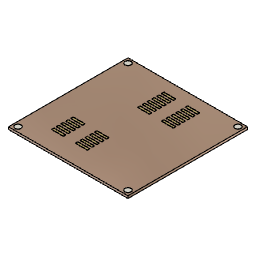
Placa v4 (Autodesk Fusion 360 design; units mm, degrees)
Autodesk Fusion 360 part; units mm, degrees
form "Form1" [no effect]
sketch "SketchPlaca" plane through (0, 0, 0) normal (0, 1, 0) x (1, 0, 0)
  line L0 (0, 0) -> (50, 0)
  line L1 (50, 0) -> (50, -50)
  line L2 (50, -50) -> (0, -50)
  line L3 (0, -50) -> (0, 0)
  dimension "d97" = 50
  dimension "d98" = 50
  constraint horizontal L0
  constraint vertical L1
  constraint horizontal L2
  constraint vertical L3
  constraint coincident L0.start L3.end
  measures "d97" distance of L0.start L0.end
  measures "d98" distance of L0.start L2.end
extrude "Extrude39" add sketch "SketchPlaca" along normal blind 1 makes body 1
sketch "SketchHoyos" plane through (0, 0, 0) normal (0, -1, 0) x (1, 0, 0)
  line L0 (50, 50) -> (0, 50)
  line L1 (0, 50) -> (0, 0)
  line L2 (0, 0) -> (50, 0)
  line L3 (50, 0) -> (50, 50)
  circle A0 centre (2, 48) radius 1.25
  circle A1 centre (2, 2) radius 1.25
  circle A2 centre (48, 2) radius 1.25
  circle A3 centre (48, 48) radius 1.25
  line L4 (1.3017, 49.0368) -> (2.7, 46.9644)
  line L5 (2.8637, 48.9036) -> (1.1304, 47.102)
  line L6 (1.1304, 2.898) -> (2.8637, 1.0964)
  line L7 (1.1827, 1.0542) -> (2.8245, 2.9395)
  line L8 (47.1174, 2.8852) -> (48.8811, 1.1134)
  line L9 (48.7554, 2.9959) -> (47.2457, 1.0032)
  line L10 (46.8338, 48.45) -> (49.1623, 47.5401)
  line L11 (48.285, 49.2171) -> (47.7194, 46.7819)
  dimension "d101" = 2.5
  dimension "d102" = 2.5
  dimension "d103" = 2.5
  dimension "d104" = 2.5
  constraint coincident A0 L4.start
  constraint coincident A0 L4.end
  constraint coincident A0 L5.start
  constraint coincident A0 L5.end
  constraint coincident A1 L6.start
  constraint coincident A1 L6.end
  constraint coincident A1 L7.start
  constraint coincident A1 L7.end
  constraint coincident A2 L8.start
  constraint coincident A2 L8.end
  constraint coincident A2 L9.start
  constraint coincident A2 L9.end
  constraint coincident A3 L10.start
  constraint coincident A3 L10.end
  constraint coincident A3 L11.start
  constraint coincident A3 L11.end
  measures "d101" diameter of A0
  measures "d102" diameter of A1
  measures "d103" diameter of A2
  measures "d104" diameter of A3
extrude "Extrude40" add sketch "SketchHoyos" along normal blind 0.1 separate body contours A0 L4 L5 | A0 L4 L5 | A0 L4 L5 | A0 L4 L5 makes body 2
extrude "Extrude41" add sketch "SketchHoyos" along normal blind 0.1 separate body contours A1 L6 L7 | A1 L6 L7 | A1 L6 L7 | A1 L6 L7 makes body 3
extrude "Extrude42" add sketch "SketchHoyos" along normal blind 0.1 separate body contours A2 L8 L9 | A2 L8 L9 | A2 L8 L9 | A2 L8 L9 makes body 4
extrude "Extrude43" add sketch "SketchHoyos" along normal blind 0.1 separate body contours A3 L10 L11 | A3 L10 L11 | A3 L10 L11 | A3 L10 L11 makes body 5
sketch "SketchPaths" plane through (0, 0, 0) normal (0, -1, 0) x (1, 0, 0)
  line L0 (50, 50) -> (0, 50)
  line L1 (0, 50) -> (0, 0)
  line L2 (0, 0) -> (50, 0)
  line L3 (50, 0) -> (50, 50)
  line L4 (10, 15) -> (15, 15)
  line L5 (15, 15) -> (15, 14)
  line L6 (15, 14) -> (10, 14)
  line L7 (10, 14) -> (10, 15)
  line L8 (10, 13) -> (15, 13)
  line L9 (15, 13) -> (15, 12)
  line L10 (15, 12) -> (10, 12)
  line L11 (10, 12) -> (10, 13)
  line L12 (10, 11) -> (15, 11)
  line L13 (15, 11) -> (15, 10)
  line L14 (15, 10) -> (10, 10)
  line L15 (10, 10) -> (10, 11)
  line L16 (10, 9) -> (15, 9)
  line L17 (15, 9) -> (15, 8)
  line L18 (15, 8) -> (10, 8)
  line L19 (10, 8) -> (10, 9)
  line L20 (10, 17) -> (15, 17)
  line L21 (15, 17) -> (15, 16)
  line L22 (15, 16) -> (10, 16)
  line L23 (10, 16) -> (10, 17)
  line L24 (20, 17) -> (25, 17)
  line L25 (25, 17) -> (25, 16)
  line L26 (25, 16) -> (20, 16)
  line L27 (20, 16) -> (20, 17)
  line L28 (20, 15) -> (25, 15)
  line L29 (25, 15) -> (25, 14)
  line L30 (25, 14) -> (20, 14)
  line L31 (20, 14) -> (20, 15)
  line L32 (20, 13) -> (25, 13)
  line L33 (25, 13) -> (25, 12)
  line L34 (25, 12) -> (20, 12)
  line L35 (20, 12) -> (20, 13)
  line L36 (20, 11) -> (25, 11)
  line L37 (25, 11) -> (25, 10)
  line L38 (25, 10) -> (20, 10)
  line L39 (20, 10) -> (20, 11)
  line L40 (20, 9) -> (25, 9)
  line L41 (25, 9) -> (25, 8)
  line L42 (25, 8) -> (20, 8)
  line L43 (20, 8) -> (20, 9)
  line L44 (20, 45) -> (25, 45)
  line L45 (25, 45) -> (25, 44)
  line L46 (25, 44) -> (20, 44)
  line L47 (20, 44) -> (20, 45)
  line L48 (20, 43) -> (25, 43)
  line L49 (25, 43) -> (25, 42)
  line L50 (25, 42) -> (20, 42)
  line L51 (20, 42) -> (20, 43)
  line L52 (20, 41) -> (25, 41)
  line L53 (25, 41) -> (25, 40)
  line L54 (25, 40) -> (20, 40)
  line L55 (20, 40) -> (20, 41)
  line L56 (20, 39) -> (25, 39)
  line L57 (25, 39) -> (25, 38)
  line L58 (25, 38) -> (20, 38)
  line L59 (20, 38) -> (20, 39)
  line L60 (20, 37) -> (25, 37)
  line L61 (25, 37) -> (25, 36)
  line L62 (25, 36) -> (20, 36)
  line L63 (20, 36) -> (20, 37)
  line L64 (20, 35) -> (25, 35)
  line L65 (25, 35) -> (25, 34)
  line L66 (25, 34) -> (20, 34)
  line L67 (20, 34) -> (20, 35)
  line L68 (30, 45) -> (35, 45)
  line L69 (35, 45) -> (35, 44)
  line L70 (35, 44) -> (30, 44)
  line L71 (30, 44) -> (30, 45)
  line L72 (30, 43) -> (35, 43)
  line L73 (35, 43) -> (35, 42)
  line L74 (35, 42) -> (30, 42)
  line L75 (30, 42) -> (30, 43)
  line L76 (30, 41) -> (35, 41)
  line L77 (35, 41) -> (35, 40)
  line L78 (35, 40) -> (30, 40)
  line L79 (30, 40) -> (30, 41)
  line L80 (30, 39) -> (35, 39)
  line L81 (35, 39) -> (35, 38)
  line L82 (35, 38) -> (30, 38)
  line L83 (30, 38) -> (30, 39)
  line L84 (30, 37) -> (35, 37)
  line L85 (35, 37) -> (35, 36)
  line L86 (35, 36) -> (30, 36)
  line L87 (30, 36) -> (30, 37)
  line L88 (30, 35) -> (35, 35)
  line L89 (35, 35) -> (35, 34)
  line L90 (35, 34) -> (30, 34)
  line L91 (30, 34) -> (30, 35)
  dimension "d114" = 1
  constraint horizontal L4
  constraint vertical L5
  constraint horizontal L6
  constraint vertical L7
  constraint horizontal L8
  constraint vertical L9
  constraint horizontal L10
  constraint vertical L11
  constraint horizontal L12
  constraint vertical L13
  constraint horizontal L14
  constraint vertical L15
  constraint horizontal L16
  constraint vertical L17
  constraint horizontal L18
  constraint vertical L19
  constraint horizontal L20
  constraint vertical L21
  constraint horizontal L22
  constraint vertical L23
  constraint horizontal L24
  constraint vertical L25
  constraint horizontal L26
  constraint vertical L27
  constraint horizontal L28
  constraint vertical L29
  constraint horizontal L30
  constraint vertical L31
  constraint horizontal L32
  constraint vertical L33
  constraint horizontal L34
  constraint vertical L35
  constraint horizontal L36
  constraint vertical L37
  constraint horizontal L38
  constraint vertical L39
  constraint horizontal L40
  constraint vertical L41
  constraint horizontal L42
  constraint vertical L43
  constraint horizontal L44
  constraint vertical L45
  constraint horizontal L46
  constraint vertical L47
  constraint horizontal L48
  constraint vertical L49
  constraint horizontal L50
  constraint vertical L51
  constraint horizontal L52
  constraint vertical L53
  constraint horizontal L54
  constraint vertical L55
  constraint horizontal L56
  constraint vertical L57
  constraint horizontal L58
  constraint vertical L59
  constraint horizontal L60
  constraint vertical L61
  constraint horizontal L62
  constraint vertical L63
  constraint horizontal L64
  constraint vertical L65
  constraint horizontal L66
  constraint vertical L67
  constraint horizontal L68
  constraint vertical L69
  constraint horizontal L70
  constraint vertical L71
  constraint horizontal L72
  constraint vertical L73
  constraint horizontal L74
  constraint vertical L75
  constraint horizontal L76
  constraint vertical L77
  constraint horizontal L78
  constraint vertical L79
  constraint horizontal L80
  constraint vertical L81
  constraint horizontal L82
  constraint vertical L83
  constraint horizontal L84
  constraint vertical L85
  constraint horizontal L86
  constraint vertical L87
  constraint horizontal L88
  constraint vertical L89
  constraint horizontal L90
  constraint vertical L91
  measures "d114" distance of L4.start L6.end
extrude "Extrude44" add sketch "SketchPaths" along normal blind 0.1 separate body contours L44 L45 L46 L47 makes body 6
extrude "Extrude45" add sketch "SketchPaths" along normal blind 0.1 separate body contours L48 L49 L50 L51 makes body 7
extrude "Extrude46" add sketch "SketchPaths" along normal blind 0.1 separate body contours L52 L53 L54 L55 makes body 8
extrude "Extrude47" add sketch "SketchPaths" along normal blind 0.1 separate body contours L56 L57 L58 L59 makes body 9
extrude "Extrude48" add sketch "SketchPaths" along normal blind 0.1 separate body contours L60 L61 L62 L63 makes body 10
extrude "Extrude49" add sketch "SketchPaths" along normal blind 0.1 separate body contours L64 L65 L66 L67 makes body 11
extrude "Extrude50" add sketch "SketchPaths" along normal blind 0.1 separate body contours L68 L69 L70 L71 makes body 12
extrude "Extrude51" add sketch "SketchPaths" along normal blind 0.1 separate body contours L72 L73 L74 L75 makes body 13
extrude "Extrude52" add sketch "SketchPaths" along normal blind 0.1 separate body contours L76 L77 L78 L79 makes body 14
extrude "Extrude53" add sketch "SketchPaths" along normal blind 0.1 separate body contours L80 L81 L82 L83 makes body 15
extrude "Extrude54" add sketch "SketchPaths" along normal blind 0.1 separate body contours L84 L85 L86 L87 makes body 16
extrude "Extrude55" add sketch "SketchPaths" along normal blind 0.1 separate body contours L88 L89 L90 L91 makes body 17
extrude "Extrude56" add sketch "SketchPaths" along normal blind 0.1 separate body contours L20 L21 L22 L23 makes body 18
extrude "Extrude57" add sketch "SketchPaths" along normal blind 0.1 separate body contours L4 L5 L6 L7 makes body 19
extrude "Extrude58" add sketch "SketchPaths" along normal blind 0.1 separate body contours L8 L9 L10 L11 makes body 20
extrude "Extrude59" add sketch "SketchPaths" along normal blind 0.1 separate body contours L12 L13 L14 L15 makes body 21
extrude "Extrude60" add sketch "SketchPaths" along normal blind 0.1 separate body contours L16 L17 L18 L19 makes body 22
extrude "Extrude61" add sketch "SketchPaths" along normal blind 0.1 separate body contours L24 L25 L26 L27 makes body 23
extrude "Extrude62" add sketch "SketchPaths" along normal blind 0.1 separate body contours L28 L29 L30 L31 makes body 24
extrude "Extrude63" add sketch "SketchPaths" along normal blind 0.1 separate body contours L32 L33 L34 L35 makes body 25
extrude "Extrude64" add sketch "SketchPaths" along normal blind 0.1 separate body contours L36 L37 L38 L39 makes body 26
extrude "Extrude65" add sketch "SketchPaths" along normal blind 0.1 separate body contours L40 L41 L42 L43 makes body 27
move_body "Move1" bodies 1 2 3 4 5 6 7 9 8 10 11 12 13 14 15 16 17 18 19 20 21 22 23 24 25 26 27 to x (1, 0, 0) y (0, 0, -1) z (0, 1, 0) at (0, 0, 0)
named bodies: "Placa", "Hoyo1", "Hoyo2", "Hoyo3", "Hoyo4", "Path11", "Path12", "Path13", "Path14", "Path15", "Path16", "Path17", "Path18", "Path19", "Path110", "Path111", "Path112", "Path21", "Path22", "Path23", "Path24", "Path25", "Path26", "Path27", "Path28", "Path29", "Path210"
